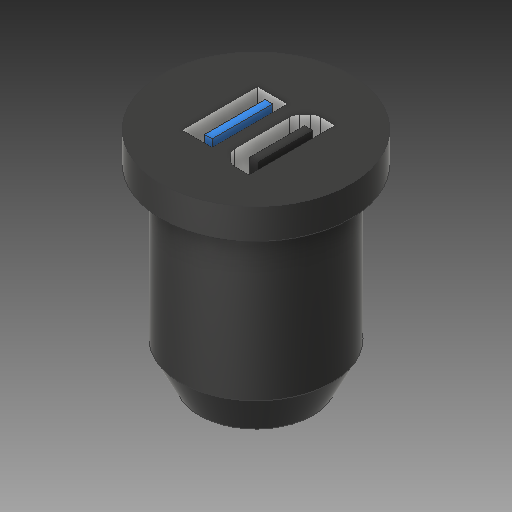
# Autodesk Inventor part: usbHdmiPanelMount
Saved by Autodesk Inventor 2018 (Build 220112000, 112)
## iProperties
Created: 2018-08-03
Part Number: usbHdmiPanelMount
Material: ABS Plastic
Document SubType Name: Modeling
Designer: Cole Tucker
Density: 1.06 g/cm^3
Appearance: Smooth - White
Mass: 19.7966 g
Surface Area: 51.2671 cm^2
Volume: 18.676 cm^3
Author: Cole Tucker
Autodesk Inventor part; units mm, degrees
ref_plane "YZ Plane" through (0, 0, 0) normal (1, 0, 0) x (0, 1, 0)
ref_plane "XZ Plane" through (0, 0, 0) normal (0, 1, 0) x (-1, 0, 0)
ref_plane "XY Plane" through (0, 0, 0) normal (0, 0, 1) x (1, 0, 0)
sketch "Sketch1" plane through (0, 0, 0) normal (0, 1, 0) x (-1, 0, 0)
  circle A0 centre (0, 0) radius 12.7
  dimension "d0" = 25.4
  constraints: 1 centre point, 1 coincident
  measures "d0" diameter of A0
extrude "Extrusion1" add sketch "Sketch1" along normal blind 25.4
sketch "Sketch2" plane through (0, 25.4, 0) normal (0, 1, 0) x (1, 0, 0)
  circle A0 centre (0, 0) radius 15.875
  dimension "d3" = 31.75
  constraints: 1 centre point, 1 coincident
  measures "d3" diameter of A0
extrude "Extrusion2" add sketch "Sketch2" along normal blind 5.08
sketch "Sketch3" plane through (0, 0, 0) normal (0, -1, 0) x (1, 0, 0)
  circle A0 centre (0, 0) radius 12.7 projected
extrude "Extrusion3" add sketch "Sketch3" along normal blind 6.35
chamfer "Chamfer1" distance 3.175 distance2 6.35 1 edges at (-12.7, -6.35, 0) measured on face at (0.3934, -6.35, -3.2397)
sketch "Sketch4" plane through (0, 30.48, 0) normal (0, 1, 0) x (1, 0, 0)
  line L0 (0, 0) -> (1.016, 0) construction
  line L1 (0, 0) -> (-1.016, 0) construction
  line L2 (-1.016, 0) -> (-3.556, 0) construction
  line L3 (-3.556, 0) -> (-3.556, 6.35) construction
  line L4 (-3.556, 6.35) -> (-1.016, 6.35) construction
  line L5 (-1.016, 6.35) -> (-1.016, 0) construction
  line L6 (-1.016, 6.35) -> (-6.096, 6.35)
  line L7 (-6.096, 6.35) -> (-6.096, -6.35)
  line L8 (-6.096, -6.35) -> (-1.016, -6.35)
  line L9 (-1.016, -6.35) -> (-1.016, 6.35)
  line L10 (1.016, 0) -> (1.016, 7.239) construction
  line L11 (1.016, 0) -> (6.096, 0) construction
  line L12 (3.556, 0) -> (3.556, 4.572) construction
  line L13 (3.556, 0) -> (3.556, -4.572) construction
  line L14 (3.556, 4.572) -> (4.826, 4.572) construction
  line L15 (3.556, -4.572) -> (2.286, -4.572) construction
  line L16 (4.826, 4.572) -> (3.556, 4.572)
  line L17 (3.556, 4.572) -> (3.556, -4.572)
  line L18 (3.556, -4.572) -> (4.826, -4.572)
  line L19 (4.826, -4.572) -> (4.826, 4.572)
  line L20 (1.016, 7.239) -> (6.096, 7.239) construction
  line L21 (6.096, 7.239) -> (3.5838, 7.239)
  line L22 (1.016, 4.6712) -> (1.016, -4.6712)
  line L23 (3.5838, -7.239) -> (6.096, -7.239)
  line L24 (6.096, -7.239) -> (6.096, 7.239)
  line L25 (-2.286, 0) -> (-3.556, 0)
  line L26 (-3.556, 0) -> (-3.556, 5.08)
  line L27 (-3.556, 5.08) -> (-2.286, 5.08)
  line L28 (-2.286, 5.08) -> (-2.286, 0)
  line L29 (-2.286, 0) -> (-3.556, 0)
  line L30 (-3.556, 0) -> (-3.556, -5.08)
  line L31 (-3.556, -5.08) -> (-2.286, -5.08)
  line L32 (-2.286, -5.08) -> (-2.286, 0)
  line L33 (1.016, 7.239) -> (1.016, 5.334) construction
  line L34 (1.016, -7.239) -> (1.016, -5.334) construction
  line L35 (1.016, -7.239) -> (2.921, -7.239) construction
  line L36 (1.016, 7.239) -> (2.921, 7.239) construction
  line L37 (2.4523, 6.7703) -> (1.4847, 5.8027)
  line L38 (1.4847, -5.8027) -> (2.4523, -6.7703)
  arc A0 (3.5838, 7.239) -> (2.4523, 6.7703) centre (3.5838, 5.6388) ccw
  arc A1 (1.4847, 5.8027) -> (1.016, 4.6712) centre (2.6162, 4.6712) ccw
  arc A2 (1.016, -4.6712) -> (1.4847, -5.8027) centre (2.6162, -4.6712) ccw
  arc A3 (2.4523, -6.7703) -> (3.5838, -7.239) centre (3.5838, -5.6388) ccw
  dimension "d11" = 1.016
  dimension "d12" = 1.016
  dimension "d13" = 2.54
  dimension "d14" = 6.35
  dimension "d15" = 5.08
  dimension "d16" = 12.7
  dimension "d17" = 7.239
  dimension "d18" = 5.08
  dimension "d19" = 4.572
  dimension "d20" = 4.572
  dimension "d21" = 1.27
  dimension "d22" = 1.27
  dimension "d23" = 5.08
  dimension "d24" = 14.478
  dimension "d25" = 5.08
  dimension "d26" = 5.08
  dimension "d27" = 1.905
  dimension "d28" = 1.905
  dimension "d29" = 1.905
  dimension "d30" = 1.905
  dimension "d31" = 1.6002
  constraints: 78 end point, 14 point on line, 12 horizontal, 12 parallel, 8 point on circle, 8 tangent, 7 perpendicular, 4 centre point, 3 equal radius, 2 midpoint, 2 vertical
  measures "d11" distance of L0.start L0.end
  measures "d12" distance of L0.start L1.end
  measures "d13" distance of L3.end L4.end
  measures "d14" distance of L2.end L3.end
  measures "d15" distance of L8.end L7.end
  measures "d16" distance of L7.end L6.end
  measures "d17" distance of L0.end L10.end
  measures "d18" distance of L0.end L11.end
  measures "d19" distance of L12.start L12.end
  measures "d20" distance of L12.start L13.end
  measures "d21" distance of L12.end L14.end
  measures "d22" distance of L13.end L15.end
  measures "d23" distance of L23.end L34.start
  measures "d24" distance of L34.start L33.start
  measures "d25" distance of L25.end L26.end
  measures "d26" distance of L30.end L29.end
  measures "d27" distance of L33.start L33.end
  measures "d28" distance of L34.start L34.end
  measures "d29" distance of L34.start L35.end
  measures "d30" distance of L33.start L36.end
  measures "d31" radius of A0
extrude "Extrusion4" cut sketch "Sketch4" against normal blind 6.35
body "Solid1"
